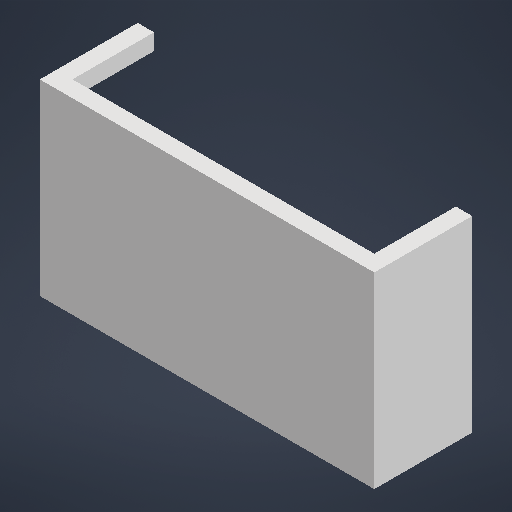
# Autodesk Inventor part: モーターホルダー試作２
Saved by Autodesk Inventor 2026 (Build 300175000, 175)
## iProperties
Created: 2025-10-26
Part Number: モーターホルダー試作２
Material: 一般
Document SubType Name: Modeling
Designer: masak
Density: 1 g/cm^3
Appearance: 既定
Author: masak
Autodesk Inventor part; units mm, degrees
ref_plane "YZ Plane" through (0, 0, 0) normal (1, 0, 0) x (0, 1, 0)
ref_plane "XZ Plane" through (0, 0, 0) normal (0, 1, 0) x (-1, 0, 0)
ref_plane "XY Plane" through (0, 0, 0) normal (0, 0, 1) x (1, 0, 0)
sketch "スケッチ2" plane through (0, 0, 0) normal (0, 0, 1) x (1, 0, 0)
  line L0 (0, 19) -> (32, 19)
  line L1 (37, 19) -> (32, 19)
  line L2 (37, 0) -> (37, 19)
  line L3 (37, 0) -> (32, 0)
  line L4 (0, 0) -> (32, 0)
  line L5 (0, 0) -> (0, 9)
  line L6 (0, 9) -> (0, 19)
  line L7 (39, 21) -> (-2, 21)
  line L8 (-2, 21) -> (-2, -2)
  line L9 (-2, -2) -> (39, -2)
  line L10 (39, -2) -> (39, 21)
  line L11 (37, 0) -> (39, 0)
  line L12 (37, 0) -> (37, -2)
  line L13 (37, 19) -> (39, 19)
  line L14 (37, 19) -> (37, 21)
  line L15 (0, 19) -> (-2, 19)
  line L16 (0, 19) -> (0, 21)
  line L17 (0, 0) -> (-2, 0)
  line L18 (0, 0) -> (0, -2)
extrude "押し出し1" add sketch "スケッチ2" against normal blind 10 contours L15 L8 L7 L16 | L13 L10 L11 L2 | L14 L7 L10 L13 | L18 L9 L8 L17 | L11 L10 L9 L12
sketch "スケッチ3" plane through (0, 0, 0) normal (0, 0, 1) x (1, 0, 0)
  line L0 (-2, 21) -> (0, 21) projected
  line L1 (39, 21) -> (39, -2) projected
  line L2 (-2, 21) -> (39, 21)
  line L3 (39, 21) -> (39, -2)
  line L4 (39, -2) -> (-2, -2)
  line L5 (-2, -2) -> (-2, 21)
  point P0 (0, 0)
  constraints: 8 end point, 2 parallel, 1 horizontal, 1 perpendicular
extrude "押し出し2" add sketch "スケッチ3" along normal blind 2
